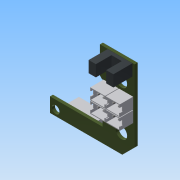
# Autodesk Inventor part: плата хотэнда
Saved by Autodesk Inventor 2017 (Build 210142000, 142)
## iProperties
Part Number: плата хотэнда
Material: Типовые
Document SubType Name: Modeling
Designer: Max
Mass: 2.53149 g
Surface Area: 44.9493 cm^2
Volume: 2.53149 cm^3
Density: 1 g/cm^3
Appearance: Темно-оливковый
Author: Max
Autodesk Inventor part; units mm, degrees
ref_plane "YZ Plane" through (0, 0, 0) normal (1, 0, 0) x (0, 1, 0)
ref_plane "XZ Plane" through (0, 0, 0) normal (0, 1, 0) x (-1, 0, 0)
ref_plane "XY Plane" through (0, 0, 0) normal (0, 0, 1) x (1, 0, 0)
sketch "Эскиз1" plane through (0, 0, 0) normal (0, 1, 0) x (-1, 0, 0)
  line L0 (6.5, 0) -> (44.45, 0)
  line L1 (44.45, 0) -> (44.45, 7.53)
  line L2 (44.45, 7.53) -> (16.84, 7.53)
  line L3 (16.84, 7.53) -> (16.84, 29.11)
  line L4 (0, 44.31) -> (0, 6.5)
  line L5 (16.84, 29.11) -> (18.22, 29.11)
  line L6 (18.22, 29.11) -> (18.22, 44.31)
  line L7 (18.22, 44.31) -> (0, 44.31)
  circle A0 centre (6.95, 33.31) radius 3
  circle A1 centre (6.95, 9.81) radius 3
  line L8 (0, 6.5) -> (6.5, 0)
  circle A2 centre (41.45, 3) radius 2
  line L9 (36.85, 7.33) -> (20.95, 7.33)
  line L10 (20.95, 7.33) -> (20.95, 0.2)
  line L11 (20.95, 0.2) -> (36.85, 0.2)
  line L12 (36.85, 0.2) -> (36.85, 7.33)
  line L13 (36.25, 6.73) -> (21.55, 6.73)
  line L14 (21.55, 6.73) -> (21.55, 0.8)
  line L15 (21.55, 0.8) -> (36.25, 0.8)
  line L16 (36.25, 0.8) -> (36.25, 6.73)
  line L17 (35.3642, 5.2366) -> (34.9642, 5.2366)
  line L18 (34.9642, 5.2366) -> (34.9642, 4.8366)
  line L19 (34.9642, 4.8366) -> (35.3642, 4.8366)
  line L20 (35.3642, 4.8366) -> (35.3642, 5.2366)
  line L21 (35.3642, 2.7366) -> (34.9642, 2.7366)
  line L22 (35.3642, 2.3366) -> (35.3642, 2.7366)
  line L23 (34.9642, 2.3366) -> (35.3642, 2.3366)
  line L24 (34.9642, 2.7366) -> (34.9642, 2.3366)
  line L25 (32.8642, 5.2366) -> (32.4642, 5.2366)
  line L26 (32.8642, 4.8366) -> (32.8642, 5.2366)
  line L27 (32.4642, 4.8366) -> (32.8642, 4.8366)
  line L28 (32.4642, 5.2366) -> (32.4642, 4.8366)
  line L29 (32.8642, 2.7366) -> (32.4642, 2.7366)
  line L30 (32.8642, 2.3366) -> (32.8642, 2.7366)
  line L31 (32.4642, 2.3366) -> (32.8642, 2.3366)
  line L32 (32.4642, 2.7366) -> (32.4642, 2.3366)
  line L33 (30.3642, 5.2366) -> (29.9642, 5.2366)
  line L34 (30.3642, 4.8366) -> (30.3642, 5.2366)
  line L35 (29.9642, 4.8366) -> (30.3642, 4.8366)
  line L36 (29.9642, 5.2366) -> (29.9642, 4.8366)
  line L37 (30.3642, 2.7366) -> (29.9642, 2.7366)
  line L38 (30.3642, 2.3366) -> (30.3642, 2.7366)
  line L39 (29.9642, 2.3366) -> (30.3642, 2.3366)
  line L40 (29.9642, 2.7366) -> (29.9642, 2.3366)
  line L41 (27.8642, 5.2366) -> (27.4642, 5.2366)
  line L42 (27.8642, 4.8366) -> (27.8642, 5.2366)
  line L43 (27.4642, 4.8366) -> (27.8642, 4.8366)
  line L44 (27.4642, 5.2366) -> (27.4642, 4.8366)
  line L45 (27.8642, 2.7366) -> (27.4642, 2.7366)
  line L46 (27.8642, 2.3366) -> (27.8642, 2.7366)
  line L47 (27.4642, 2.3366) -> (27.8642, 2.3366)
  line L48 (27.4642, 2.7366) -> (27.4642, 2.3366)
  line L49 (25.3642, 5.2366) -> (24.9642, 5.2366)
  line L50 (25.3642, 4.8366) -> (25.3642, 5.2366)
  line L51 (24.9642, 4.8366) -> (25.3642, 4.8366)
  line L52 (24.9642, 5.2366) -> (24.9642, 4.8366)
  line L53 (25.3642, 2.7366) -> (24.9642, 2.7366)
  line L54 (25.3642, 2.3366) -> (25.3642, 2.7366)
  line L55 (24.9642, 2.3366) -> (25.3642, 2.3366)
  line L56 (24.9642, 2.7366) -> (24.9642, 2.3366)
  line L57 (22.8642, 5.2366) -> (22.4642, 5.2366)
  line L58 (22.8642, 4.8366) -> (22.8642, 5.2366)
  line L59 (22.4642, 4.8366) -> (22.8642, 4.8366)
  line L60 (22.4642, 5.2366) -> (22.4642, 4.8366)
  line L61 (22.8642, 2.7366) -> (22.4642, 2.7366)
  line L62 (22.8642, 2.3366) -> (22.8642, 2.7366)
  line L63 (22.4642, 2.3366) -> (22.8642, 2.3366)
  line L64 (22.4642, 2.7366) -> (22.4642, 2.3366)
  point P0 (0, 0)
  dimension "d2" = 16.84
  dimension "d3" = 18.22
  dimension "d5" = 7.53
  dimension "d6" = 6
  dimension "d7" = 6
  dimension "d8" = 23.5
  dimension "d10" = 44.45
  dimension "d11" = 44.45
  dimension "d13" = 45
  dimension "d14" = 6.5
  dimension "d15" = 3.95
  dimension "d17" = 4
  dimension "d18" = 1
  dimension "d19" = 1
  dimension "d20" = 0.2
  dimension "d21" = 0.2
  dimension "d22" = 7.6
  dimension "d23" = 15.9
  dimension "d24" = 0.6
  dimension "d25" = 0.6
  dimension "d26" = 0.6
  dimension "d27" = 0.6
  dimension "d28" = 0.4
  dimension "d29" = 0.4
  dimension "d32" = 2.5
  dimension "d35" = 2.5
  dimension "d38" = 11
  dimension "d39" = 44.31
  dimension "d40" = 44.31
  dimension "d41" = 6.95
  dimension "d42" = 9.81
  constraints: 130 end point, 9 parallel, 6 horizontal, 5 perpendicular, 3 centre point, 1 vertical, 88 other
  measures "d2" distance between parallel lines of L4 L3
  measures "d3" distance between parallel lines of L4 L6
  measures "d5" distance between parallel lines of L0 L2
  measures "d6" diameter of A0
  measures "d7" diameter of A1
  measures "d8" distance of A0.centre A1.centre
  measures "d10" distance between parallel lines of L4 L1
  measures "d11" distance from line of point (0, 0) L1
  measures "d13" angle of L4 L8
  measures "d14" distance of L0.start point (0, 0)
  measures "d15" distance edge to line of A1 L4
  measures "d17" diameter of A2
  measures "d18" distance edge to line of A2 L1
  measures "d19" distance edge to line of A2 L0
  measures "d20" distance between parallel lines of L2 L9
  measures "d21" distance between parallel lines of L0 L11
  measures "d22" distance between parallel lines of L1 L12
  measures "d23" distance between parallel lines of L10 L12
  measures "d24" distance between parallel lines of L9 L13
  measures "d25" distance between parallel lines of L11 L15
  measures "d26" distance between parallel lines of L12 L16
  measures "d27" distance between parallel lines of L10 L14
  measures "d28" distance of L19.end L18.end
  measures "d29" distance of L18.end L17.end
  measures "d32" distance of L17.end L21.end
  measures "d35" distance of L17.end L25.end
  measures "d38" distance from line of A0.centre L7
  measures "d39" distance from line of point (0, 0) L7
  measures "d40" distance between parallel lines of L7 L0
  measures "d41" horizontal distance of point (0, 0) A1.centre
  measures "d42" vertical distance of point (0, 0) A1.centre
extrude "Выдавливание1" add sketch "Эскиз1" against normal blind 1.56 contours L8 L4 L7 L6 L5 L3 L2 L1 L0 | L12 L11 L10 L9 | L16 L15 L14 L13 | L20 L19 L18 L17 | L22 L23 L24 L21 | L26 L27 L28 L25 | L30 L31 L32 L29 | L34 L35 L36 L33 | L38 L39 L40 L37 | L42 L43 L44 L41 | L46 L47 L48 L45 | L50 L51 L52 L49 | L54 L55 L56 L53 | L58 L59 L60 L57 | L62 L63 L64 L61
extrude "Выдавливание2" add sketch "Эскиз1" along normal blind 0.5 contours L16 L15 L14 L13
extrude "Выдавливание3" add sketch "Эскиз1" along normal blind 6 contours L12 L11 L10 L9 | L20 L19 L18 L17 | L22 L23 L24 L21 | L26 L27 L28 L25 | L30 L31 L32 L29 | L34 L35 L36 L33 | L38 L39 L40 L37 | L42 L43 L44 L41 | L46 L47 L48 L45 | L50 L51 L52 L49 | L54 L55 L56 L53 | L58 L59 L60 L57 | L62 L63 L64 L61
chamfer "Фаска1" distance 1 angle 45 1 edges at (-18.22, -0.78, 29.11)
sketch "Эскиз2" plane through (0, -1.56, 0) normal (0, -1, 0) x (1, 0, 0)
  line L0 (-1.16, 44.21) -> (-14.16, 44.21)
  line L1 (-14.16, 44.21) -> (-14.16, 38.21)
  line L2 (-14.16, 38.21) -> (-1.16, 38.21)
  line L3 (-1.16, 38.21) -> (-1.16, 44.21)
  line L4 (-1.16, 44.21) -> (-4.96, 44.21)
  line L5 (-4.96, 44.21) -> (-4.96, 38.21)
  line L6 (-4.96, 38.21) -> (-1.16, 38.21)
  line L7 (-1.16, 38.21) -> (-1.16, 44.21)
  line L8 (-14.16, 44.21) -> (-10.36, 44.21)
  line L9 (-10.36, 44.21) -> (-10.36, 38.21)
  line L10 (-10.36, 38.21) -> (-14.16, 38.21)
  line L11 (-14.16, 38.21) -> (-14.16, 44.21)
  line L12 (0, 44.31) -> (-18.22, 44.31) projected
  line L13 (0, 6.5) -> (0, 44.31) projected
  line L14 (-4.96, 44.21) -> (-10.36, 44.21)
  line L15 (-10.36, 44.21) -> (-10.36, 38.21)
  line L16 (-10.36, 38.21) -> (-4.96, 38.21)
  line L17 (-4.96, 38.21) -> (-4.96, 44.21)
  point P0 (0, 0)
  dimension "d52" = 6
  dimension "d53" = 13
  dimension "d54" = 0.1
  dimension "d55" = 1.16
  dimension "d56" = 3.8
  dimension "d57" = 3.8
  constraints: 32 end point, 8 parallel, 4 horizontal, 4 perpendicular, 2 point on line
  measures "d52" distance between parallel lines of L2 L0
  measures "d53" distance between parallel lines of L1 L3
  measures "d54" distance between parallel lines of L12 L0
  measures "d55" distance between parallel lines of L3 L13
  measures "d56" distance between parallel lines of L5 L3
  measures "d57" distance between parallel lines of L1 L9
extrude "Выдавливание4" add sketch "Эскиз2" along normal blind 1.8
extrude "Выдавливание5" add sketch "Эскиз2" along normal blind 10 contours L3 L2 L5 L0 | L9 L2 L1 L0
sketch "Эскиз3" plane through (0, -1.56, 0) normal (0, -1, 0) x (1, 0, 0)
  line L0 (-10.36, 38.21) -> (-4.96, 38.21) construction
  line L1 (-16.84, 29.11) -> (-16.84, 7.53) construction
  line L2 (0, 6.5) -> (0, 44.31) construction
  line L3 (-16.34, 29.21) -> (-8.5, 29.21)
  line L4 (-8.5, 29.21) -> (-8.5, 23.36)
  line L5 (-8.5, 23.36) -> (-16.34, 23.36)
  line L6 (-16.34, 23.36) -> (-16.34, 29.21)
  line L7 (-0.8, 29.21) -> (-8.2, 29.21)
  line L8 (-8.2, 29.21) -> (-8.2, 23.36)
  line L9 (-8.2, 23.36) -> (-0.8, 23.36)
  line L10 (-0.8, 23.36) -> (-0.8, 29.21)
  line L11 (-16.34, 17.21) -> (-8.5, 17.21)
  line L12 (-8.5, 17.21) -> (-8.5, 23.06)
  line L13 (-8.5, 23.06) -> (-16.34, 23.06)
  line L14 (-16.34, 23.06) -> (-16.34, 17.21)
  line L15 (-8.2, 23.06) -> (-0.8, 23.06)
  line L16 (-0.8, 23.06) -> (-0.8, 17.21)
  line L17 (-0.8, 17.21) -> (-8.2, 17.21)
  line L18 (-8.2, 17.21) -> (-8.2, 23.06)
  line L19 (-8.9, 28.81) -> (-15.94, 28.81)
  line L20 (-15.94, 28.81) -> (-15.94, 23.76)
  line L21 (-15.94, 23.76) -> (-8.9, 23.76)
  line L22 (-8.9, 23.76) -> (-8.9, 28.81)
  line L23 (-7.8, 28.81) -> (-1.2, 28.81)
  line L24 (-1.2, 28.81) -> (-1.2, 23.76)
  line L25 (-1.2, 23.76) -> (-7.8, 23.76)
  line L26 (-7.8, 23.76) -> (-7.8, 28.81)
  line L27 (-1.2, 22.66) -> (-7.8, 22.66)
  line L28 (-7.8, 22.66) -> (-7.8, 17.61)
  line L29 (-7.8, 17.61) -> (-1.2, 17.61)
  line L30 (-1.2, 17.61) -> (-1.2, 22.66)
  line L31 (-15.94, 22.66) -> (-8.9, 22.66)
  line L32 (-8.9, 22.66) -> (-8.9, 17.61)
  line L33 (-8.9, 17.61) -> (-15.94, 17.61)
  line L34 (-15.94, 17.61) -> (-15.94, 22.66)
  line L35 (-14.5197, 20.5794) -> (-13.6821, 20.5794)
  line L36 (-13.6821, 20.5794) -> (-13.6821, 20.0347)
  line L37 (-13.6821, 20.0347) -> (-14.5197, 20.0347)
  line L38 (-14.5197, 20.0347) -> (-14.5197, 20.5794)
  line L39 (-11.2982, 20.5794) -> (-10.4603, 20.5794)
  line L40 (-10.4603, 20.5794) -> (-10.4603, 20.0347)
  line L41 (-10.4603, 20.0347) -> (-11.2982, 20.0347)
  line L42 (-11.2982, 20.0347) -> (-11.2982, 20.5794)
  line L43 (-14.5197, 26.5794) -> (-13.6821, 26.5794)
  line L44 (-14.5197, 26.0347) -> (-14.5197, 26.5794)
  line L45 (-13.6821, 26.5794) -> (-13.6821, 26.0347)
  line L46 (-11.2982, 26.5794) -> (-10.4603, 26.5794)
  line L47 (-11.2982, 26.0347) -> (-11.2982, 26.5794)
  line L48 (-10.4603, 26.5794) -> (-10.4603, 26.0347)
  line L49 (-10.4603, 26.0347) -> (-11.2982, 26.0347)
  line L50 (-13.6821, 26.0347) -> (-14.5197, 26.0347)
  line L51 (-6.5197, 20.5794) -> (-5.6821, 20.5794)
  line L52 (-6.5197, 20.0347) -> (-6.5197, 20.5794)
  line L53 (-5.6821, 20.5794) -> (-5.6821, 20.0347)
  line L54 (-3.2982, 20.5794) -> (-2.4603, 20.5794)
  line L55 (-3.2982, 20.0347) -> (-3.2982, 20.5794)
  line L56 (-2.4603, 20.5794) -> (-2.4603, 20.0347)
  line L57 (-2.4603, 20.0347) -> (-3.2982, 20.0347)
  line L58 (-5.6821, 20.0347) -> (-6.5197, 20.0347)
  line L59 (-6.5197, 26.5794) -> (-5.6821, 26.5794)
  line L60 (-6.5197, 26.0347) -> (-6.5197, 26.5794)
  line L61 (-5.6821, 26.5794) -> (-5.6821, 26.0347)
  line L62 (-3.2982, 26.5794) -> (-2.4603, 26.5794)
  line L63 (-3.2982, 26.0347) -> (-3.2982, 26.5794)
  line L64 (-2.4603, 26.5794) -> (-2.4603, 26.0347)
  line L65 (-2.4603, 26.0347) -> (-3.2982, 26.0347)
  line L66 (-5.6821, 26.0347) -> (-6.5197, 26.0347)
  point P0 (0, 0)
  dimension "d66" = 0.3
  dimension "d67" = 0.3
  dimension "d68" = 15.54
  dimension "d70" = 0.4
  dimension "d71" = 0.4
  dimension "d72" = 0.4
  dimension "d73" = 0.4
  dimension "d76" = 6
  dimension "d79" = 8
  constraints: 128 end point, 20 parallel, 12 point on line, 10 perpendicular, 7 horizontal, 1 vertical, 60 other
  measures "d66" distance between parallel lines of L13 L5
  measures "d67" distance between parallel lines of L8 L4
  measures "d68" distance between parallel lines of L6 L10
  measures "d70" distance between parallel lines of L3 L19
  measures "d71" distance between parallel lines of L7 L23
  measures "d72" distance between parallel lines of L15 L27
  measures "d73" distance between parallel lines of L13 L31
  measures "d76" distance of L35.end L43.end
  measures "d79" distance of L35.end L51.end
extrude "Выдавливание6" add sketch "Эскиз3" along normal blind 7
extrude "Выдавливание7" add sketch "Эскиз3" along normal blind 1 contours L22 L21 L20 L19 | L23 L24 L25 L26 | L30 L29 L28 L27 | L31 L32 L33 L34
sketch "Эскиз4" plane through (0, -8.56, 0) normal (0, -1, 0) x (1, 0, 0)
  line L0 (-20.3543, 27.6277) -> (1.2524, 27.6277)
  line L1 (1.2524, 27.6277) -> (1.2524, 25.2131)
  line L2 (1.2524, 25.2131) -> (-20.3543, 25.2131)
  line L3 (-20.3543, 25.2131) -> (-20.3543, 27.6277)
  line L4 (-20.3543, 21.4663) -> (2.5013, 21.4663)
  line L5 (2.5013, 21.4663) -> (2.5013, 19.01)
  line L6 (2.5013, 19.01) -> (-20.3543, 19.01)
  line L7 (-20.3543, 19.01) -> (-20.3543, 21.4663)
  point P0 (0, 0)
  constraints: 16 end point, 4 parallel, 2 horizontal, 2 perpendicular, 1 point on line
extrude "Выдавливание8" cut sketch "Эскиз4" against normal blind 1.5
